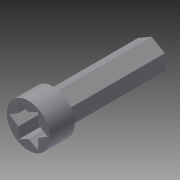
# Autodesk Inventor part: 000111
Saved by Autodesk Inventor 2015 (Build 190159000, 159)
## iProperties
Created: 2015-05-18
Part Number: 000111
Material: Generic
Document SubType Name: Modeling
Designer: Wesley
Density: 1 g/cm^3
Appearance: Default
Author: Wesley
Autodesk Inventor part; units mm, degrees
ref_plane "YZ Plane" through (0, 0, 0) normal (1, 0, 0) x (0, 1, 0)
ref_plane "XZ Plane" through (0, 0, 0) normal (0, 1, 0) x (-1, 0, 0)
ref_plane "XY Plane" through (0, 0, 0) normal (0, 0, 1) x (1, 0, 0)
sketch "Sketch1" plane through (0, 0, 0) normal (0, 0, 1) x (1, 0, 0)
  line L0 (0, 3.175) -> (2.7496, 1.5875)
  line L1 (2.7496, 1.5875) -> (2.7496, -1.5875)
  line L2 (2.7496, -1.5875) -> (0, -3.175)
  line L3 (0, -3.175) -> (-2.7496, -1.5875)
  line L4 (-2.7496, -1.5875) -> (-2.7496, 1.5875)
  line L5 (-2.7496, 1.5875) -> (0, 3.175)
  point P0 (0, 0)
  point P1 (0, 0)
  dimension "d0" = 6.35
  dimension "d1" = 2.7496
  constraints: 12 end point, 1 coincident, 13 other
  measures "d0" distance of L2.end L0.start
  measures "d1" horizontal distance of L0.start L0.end
extrude "Extrusion1" add sketch "Sketch1" along normal blind 25.4
sketch "Sketch2" plane through (0, 0, 25.4) normal (0, 0, 1) x (1, 0, 0)
  circle A0 centre (0, 0) radius 4.445
  dimension "d4" = 8.89
  constraints: 1 centre point, 1 coincident
  measures "d4" diameter of A0
extrude "Extrusion2" add sketch "Sketch2" against normal blind 5.08
sketch "Sketch3" plane through (0, 0, 25.4) normal (0, 0, 1) x (1, 0, 0)
  circle A0 centre (0, 0) radius 3.9751 construction
  circle A1 centre (0, 0) radius 2.3813 construction
  line L0 (-5.2785, 0) -> (7.6367, 0) construction
  line L1 (2.0622, 1.1906) -> (3.9751, 0)
  line L2 (3.9751, 0) -> (2.0622, -1.1906)
  line L3 (2.0622, -1.1906) -> (2.0622, 1.1906)
  line L4 (0, 2.3813) -> (1.9876, 3.4425)
  line L5 (1.9876, 3.4425) -> (2.0622, 1.1906)
  line L6 (2.0622, 1.1906) -> (0, 2.3813)
  line L7 (-2.0622, 1.1906) -> (-1.9875, 3.4425)
  line L8 (-1.9875, 3.4425) -> (0, 2.3812)
  line L9 (0, 2.3812) -> (-2.0622, 1.1906)
  line L10 (-2.0622, -1.1906) -> (-3.9751, 0)
  line L11 (-3.9751, 0) -> (-2.0622, 1.1906)
  line L12 (-2.0622, 1.1906) -> (-2.0622, -1.1906)
  line L13 (0, -2.3813) -> (-1.9876, -3.4425)
  line L14 (-1.9876, -3.4425) -> (-2.0622, -1.1906)
  line L15 (-2.0622, -1.1906) -> (0, -2.3813)
  line L16 (2.0622, -1.1906) -> (1.9875, -3.4425)
  line L17 (1.9875, -3.4425) -> (0, -2.3813)
  line L18 (0, -2.3813) -> (2.0622, -1.1906)
  dimension "d7" = 7.9502
  dimension "d8" = 4.7625
  dimension "d9" = 2.0216
  dimension "d10" = 60
  dimension "d11" = 2.3813
  dimension "d14" = 360
  constraints: 38 end point, 3 coincident, 2 point on line, 1 centre point, 1 horizontal, 1 horizontal alignment, 41 other
  measures "d8" diameter of A1
  measures "d9" distance from line of L1 L2.end
  measures "d11" distance of L2.end L1.start
extrude "Extrusion3" cut sketch "Sketch3" against normal blind 4.445 contours L1 L2 L3 | L6 L4 L5 | L16 L17 L18 | L9 L7 L8 | L13 L14 L15 | L12 L10 L11
sketch "Sketch4" plane through (0, 0, 25.4) normal (0, 0, 1) x (1, 0, 0)
  line L0 (2.0622, 1.1906) -> (0, 2.3812) projected
  line L1 (0, 2.3812) -> (-2.0622, 1.1906) projected
  line L2 (-2.0622, 1.1906) -> (-2.0622, -1.1906) projected
  line L3 (-2.0622, -1.1906) -> (0, -2.3813) projected
  line L4 (0, -2.3813) -> (2.0622, -1.1906) projected
  line L5 (2.0622, -1.1906) -> (2.0622, 1.1906) projected
  point P0 (0, 0)
extrude "Extrusion4" cut sketch "Sketch4" against normal blind 4.445
body "Solid1"
